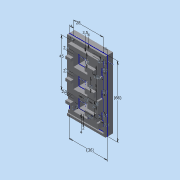
# Autodesk Inventor part: Top_V3
Saved by Autodesk Inventor 2015 (Build 190159000, 159)
## iProperties
Created: 2015-01-31
Part Number: Top_V3
Material: Generic
Document SubType Name: Modeling
Designer: Openlab
Density: 1 g/cm^3
Appearance: Default
Author: Openlab
Autodesk Inventor part; units mm, degrees
ref_plane "YZ Plane" through (0, 0, 0) normal (1, 0, 0) x (0, 1, 0)
ref_plane "XZ Plane" through (0, 0, 0) normal (0, 1, 0) x (-1, 0, 0)
ref_plane "XY Plane" through (0, 0, 0) normal (0, 0, 1) x (1, 0, 0)
sketch "Sketch1" plane through (0, 0, 0) normal (0, 1, 0) x (-1, 0, 0)
  line L0 (23, -43.5) -> (23, -56.5)
  line L1 (28, -33.25) -> (23, -33.25)
  line L2 (28, -30.75) -> (23, -30.75)
  line L3 (28, -48.75) -> (23, -48.75)
  line L4 (10, -56.5) -> (23, -56.5)
  line L5 (10, -7.5) -> (10, -20.5)
  line L6 (23, -43.5) -> (10, -43.5)
  line L7 (10, -43.5) -> (10, -56.5)
  line L8 (10, -38.5) -> (23, -38.5)
  line L9 (23, -38.5) -> (23, -25.5)
  line L10 (25.5, 0.6818) -> (25.5, -55.6748) construction
  line L11 (16.5, 0.1481) -> (16.5, -50.7513) construction
  line L12 (10, -25.5) -> (10, -38.5)
  line L13 (32.1467, -32) -> (-0.6768, -32) construction
  line L14 (10, -20.5) -> (23, -20.5)
  line L15 (23, -25.5) -> (10, -25.5)
  line L16 (23, -7.5) -> (10, -7.5)
  line L17 (30.1668, -14) -> (1.95, -14) construction
  line L18 (1.5, -34.25) -> (10, -34.25)
  line L19 (1.6727, -50) -> (31.8542, -50) construction
  line L20 (28, -60) -> (0, -60)
  line L21 (23, -51.25) -> (28, -51.25)
  line L22 (23, -7.5) -> (23, -20.5)
  line L23 (0, -29.75) -> (10, -29.75)
  line L24 (23, -15.25) -> (28, -15.25)
  line L25 (23, -12.75) -> (28, -12.75)
  line L26 (1.5, -16.25) -> (10, -16.25)
  line L27 (0, -11.75) -> (10, -11.75)
  line L28 (0, -47.75) -> (10, -47.75)
  line L29 (1.5, -52.25) -> (10, -52.25)
  line L30 (28, 0) -> (0, 0)
  line L31 (28, 0) -> (32, 0)
  line L32 (32, 0) -> (32, -66)
  line L33 (32, -66) -> (-4, -66)
  line L34 (-4, -66) -> (-4, 0)
  line L35 (28, -5) -> (30, -5)
  line L36 (30, -5) -> (30, -50)
  line L37 (30, -50) -> (32, -50)
  line L38 (-4, 0) -> (0, 0)
  line L39 (0, -5) -> (-2, -5)
  line L40 (-2, -5) -> (-2, -64)
  line L41 (-2, -64) -> (32, -64)
  line L42 (28, -4) -> (0, -4)
  line L43 (38, -5) -> (-10, -5) construction
  line L44 (0, -60) -> (0, -55.25)
  line L45 (0, -47.75) -> (0, -37.25)
  line L46 (0, -29.75) -> (0, -19.25)
  line L47 (0, -11.75) -> (0, 0)
  line L48 (1.5, -11.75) -> (1.5, -16.25)
  line L49 (1.5, -29.75) -> (1.5, -34.25)
  line L50 (1.5, -47.75) -> (1.5, -52.25)
  line L51 (1.5, -52.25) -> (1.5, -55.25)
  line L52 (1.5, -55.25) -> (0, -55.25)
  line L53 (1.5, -34.25) -> (1.5, -37.25)
  line L54 (1.5, -37.25) -> (0, -37.25)
  line L55 (1.5, -16.25) -> (1.5, -19.25)
  line L56 (1.5, -19.25) -> (0, -19.25)
  line L57 (28, 0) -> (28, -5)
  line L58 (31, -55.625) -> (29, -55.625) construction
  line L59 (28, -53.625) -> (26.5, -53.625)
  line L60 (26.5, -53.625) -> (26.5, -57.625)
  line L61 (26.5, -57.625) -> (28, -57.625)
  line L62 (28, -5) -> (28, -53.625)
  line L63 (28, -57.625) -> (28, -60)
  point P0 (16.5, -14)
  point P1 (16.5, -32)
  point P2 (16.5, -50)
  dimension "d0" = 13
  dimension "d3" = 2.5
  dimension "d6" = 4.5
  dimension "d7" = 4.5
  dimension "d8" = 4.5
  dimension "d10" = 13
  dimension "d11" = 18
  dimension "d12" = 18
  dimension "d13" = 13
  dimension "d16" = 13
  dimension "d17" = 3.5
  dimension "d18" = 4
  dimension "d20" = 45
  dimension "d21" = 4
  dimension "d22" = 2
  dimension "d23" = 2.5
  dimension "d24" = 3.5
  dimension "d25" = 4
  dimension "d26" = 2.5
  dimension "d27" = 2
  dimension "d28" = 4
  dimension "d29" = 66
  dimension "d30" = 36
  dimension "d37" = 1.5
  dimension "d38" = 10
  dimension "d39" = 2.5
  dimension "d55" = 3
  dimension "d58" = 28
  dimension "d59" = 2
  dimension "d60" = 1.5
  dimension "d61" = 4
  constraints: 128 end point, 39 point on line, 27 perpendicular, 14 collinear, 13 horizontal, 7 vertical, 6 parallel, 2 coincident, 12 other
  measures "d0" distance of L0.end L0.start
  measures "d3" distance between parallel lines of L2 L1
  measures "d6" distance between parallel lines of L27 L26
  measures "d7" distance between parallel lines of L23 L18
  measures "d8" distance between parallel lines of L29 L28
  measures "d10" distance between parallel lines of L14 L16
  measures "d11" distance between parallel lines of L13 L17
  measures "d12" distance between parallel lines of L19 L13
  measures "d13" distance between parallel lines of L7 L0
  measures "d16" distance between parallel lines of L8 L15
  measures "d17" distance between parallel lines of L20 L4
  measures "d18" distance of L30.start L31.end
  measures "d20" distance of L35.end L36.end
  measures "d21" distance of L34.end L30.end
  measures "d22" distance of L39.start L39.end
  measures "d23" distance between parallel lines of L21 L3
  measures "d24" distance between parallel lines of L42 L16
  measures "d25" distance between parallel lines of L41 L20
  measures "d26" distance between parallel lines of L16 L43
  measures "d27" distance between parallel lines of L33 L41
  measures "d28" distance between parallel lines of L30 L42
  measures "d29" distance of L33.end L34.end
  measures "d30" distance of L32.end L33.end
  measures "d37" distance between parallel lines of L44 L50
  measures "d38" distance between parallel lines of L46 L5
  measures "d39" distance between parallel lines of L24 L25
  measures "d55" distance of L29.start L51.end
  measures "d58" distance between parallel lines of L57 L47
  measures "d59" distance of L35.start L35.end
  measures "d60" distance of L60.end L61.end
  measures "d61" distance of L59.end L60.end
extrude "Extrusion1" add sketch "Sketch1" against normal blind 2 contours L57 L31 L32 L37 L36 L35 | L42 L47 L30 L57 | L47 L39 L40 L41 L32 L33 L34 L38
extrude "Extrusion4" add sketch "Sketch1" against normal blind 7.5 contours L3 L62 L21 L0 | L7 L29 L50 L28 | L1 L9 L2 L62 | L24 L22 L25 L62 | L18 L49 L23 L12 | L26 L48 L27 L5
extrude "Extrusion5" add sketch "Sketch1" against normal blind 5 contours L6 L7 L28 L45 L54 L53 L18 L12 L8 L9 L1 L62 L3 L0 | L21 L62 L59 L60 L61 L63 L20 L44 L52 L51 L29 L7 L4 L0 | L2 L9 L15 L12 L23 L46 L56 L55 L26 L5 L14 L22 L24 L62 | L25 L22 L16 L5 L27 L47 L42 L57 L62
extrude "Extrusion6" add sketch "Sketch1" along normal blind 5 contours L6 L7 L28 L45 L54 L53 L18 L12 L8 L9 L1 L62 L3 L0 | L3 L62 L21 L0 | L21 L62 L59 L60 L61 L63 L20 L44 L52 L51 L29 L7 L4 L0 | L62 L35 L36 L37 L32 L41 L40 L39 L47 L27 L48 L55 L56 L46 L23 L49 L53 L54 L45 L28 L50 L51 L52 L44 L20 L63 L61 L60 L59 | L7 L29 L50 L28 | L1 L9 L2 L62 | L2 L9 L15 L12 L23 L46 L56 L55 L26 L5 L14 L22 L24 L62 | L24 L22 L25 L62 | L25 L22 L16 L5 L27 L47 L42 L57 L62 | L18 L49 L23 L12 | L57 L31 L32 L37 L36 L35 | L42 L47 L30 L57 | L26 L48 L27 L5 | L47 L39 L40 L41 L32 L33 L34 L38
sketch "Sketch2" plane through (0, 5, 0) normal (0, 1, 0) x (1, 0, 0)
  line L0 (-25, 3) -> (-3, 3)
  line L1 (1, 7) -> (1, 57)
  line L2 (-3, 61) -> (-25, 61)
  line L3 (-29, 57) -> (-29, 7)
  line L4 (-32, 66) -> (-32, 0) projected
  line L5 (-32, 0) -> (4, 0) projected
  line L6 (4, 0) -> (4, 66) projected
  line L7 (4, 66) -> (-32, 66) projected
  arc A0 (-29, 7) -> (-25, 3) centre (-25, 7) ccw
  arc A1 (-25, 61) -> (-29, 57) centre (-25, 57) ccw
  arc A2 (-3, 3) -> (1, 7) centre (-3, 7) ccw
  arc A3 (1, 57) -> (-3, 61) centre (-3, 57) ccw
  point P0 (0, 0)
  dimension "d46" = 3
  dimension "d47" = 3
  dimension "d48" = 3
  dimension "d49" = 5
  dimension "d54" = 8
  constraints: 8 end point, 8 point on circle, 8 tangent, 4 centre point, 2 horizontal alignment, 2 parallel, 1 horizontal, 1 perpendicular, 1 vertical alignment
  measures "d46" distance between parallel lines of L4 L3
  measures "d47" distance between parallel lines of L5 L0
  measures "d48" distance between parallel lines of L6 L1
  measures "d49" distance between parallel lines of L7 L2
  measures "d54" diameter of A0
extrude "Extrusion7" add sketch "Sketch2" along normal blind 3 contours A0 L3 A1 L2 A3 L1 A2 L0
extrude "Extrusion8" cut sketch "Sketch1" along normal blind 10 contours L0 L4 L7 L6 | L9 L8 L12 L15 | L22 L14 L5 L16
body "Solid1"
